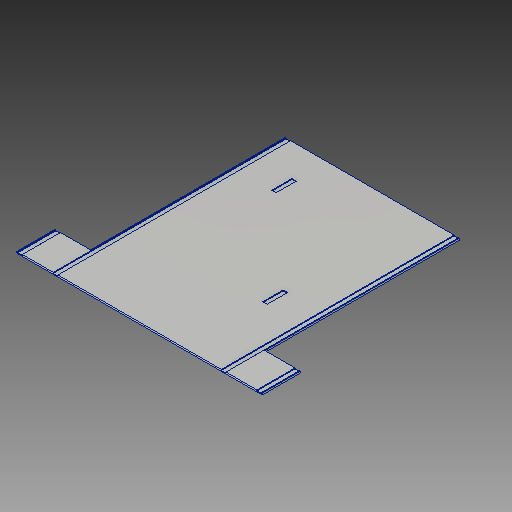
# Autodesk Inventor part: 밑판
Saved by Autodesk Inventor 2017 (Build 210142000, 142)
## iProperties
Part Number: 밑판
Material: 알루미늄 6061
Document SubType Name: Modeling
Designer: minom
Density: 2.7 g/cm^3
Appearance: 알루미늄 - 평지
Mass: 316.314 g
Surface Area: 1244.74 cm^2
Volume: 117.153 cm^3
Author: minom
Autodesk Inventor part; units mm, degrees
ref_plane "YZ Plane" through (0, 0, 0) normal (1, 0, 0) x (0, 1, 0)
ref_plane "XZ Plane" through (0, 0, 0) normal (0, 1, 0) x (-1, 0, 0)
ref_plane "XY Plane" through (0, 0, 0) normal (0, 0, 1) x (1, 0, 0)
sketch "스케치1" plane through (0, 0, 0) normal (0, 1, 0) x (-1, 0, 0)
  line L0 (-43, 66) -> (-249, 66)
  line L1 (-249, 66) -> (-249, -209)
  line L2 (-249, -209) -> (-43, -209)
  line L3 (-43, -209) -> (-43, 66)
  point P0 (0, 0)
  dimension "d0" = 206
  dimension "d1" = 275
  constraints: 8 end point, 2 parallel, 1 horizontal, 1 perpendicular
  measures "d0" distance of L2.end L1.end
  measures "d1" distance of L1.end L0.end
extrude "돌출1" add sketch "스케치1" along normal blind 2
sketch "스케치2" plane through (0, 2, 0) normal (0, 1, 0) x (1, 0, 0)
  line L0 (43, -66) -> (249, -66) projected
  line L1 (249, -66) -> (248, -66)
  line L2 (248, -66) -> (248, 209)
  line L3 (249, 209) -> (43, 209) projected
  line L4 (43, 209) -> (43, -66) projected
  line L5 (43, -66) -> (44, -66)
  line L6 (44, -66) -> (44, 209)
  line L7 (44, 209) -> (49.4, 209)
  line L8 (49.4, 209) -> (49.4, -66)
  line L9 (248, -66) -> (242.6, -66)
  line L10 (242.6, -66) -> (242.6, 209)
  line L11 (49.4, -66) -> (44, -66)
  line L12 (49.4, 209) -> (44, 209)
  point P0 (0, 0)
  dimension "d4" = 1
  dimension "d5" = 5.4
  dimension "d6" = 5.4
  dimension "d9" = 1
  constraints: 20 end point, 6 point on line, 5 perpendicular, 2 collinear
  measures "d4" distance of L0.end L1.end
  measures "d5" distance of L6.end L7.end
  measures "d6" distance of L1.end L9.end
  measures "d9" distance between parallel lines of L6 L4
extrude "돌출2" cut sketch "스케치2" against normal blind 1 contours L6 L3 L8 L0 | L10 L3 L2 L0
sketch "스케치3" plane through (0, 2, 0) normal (0, 1, 0) x (1, 0, 0)
  line L0 (197.8, 27.6733) -> (203, 27.6733)
  line L1 (203, 27.6733) -> (203, 51.8733)
  line L2 (203, 51.8733) -> (197.8, 51.8733)
  line L3 (197.8, 51.8733) -> (197.8, 27.6733)
  point P0 (0, 0)
  dimension "d10" = 5.2
  dimension "d11" = 24.2
  constraints: 8 end point, 2 parallel, 1 horizontal, 1 perpendicular, 1 other
  measures "d10" distance of L0.start L0.end
  measures "d11" distance of L0.end L1.end
extrude "돌출3" cut sketch "스케치3" against normal blind 1
sketch "스케치4" plane through (0, 2, 0) normal (0, 1, 0) x (1, 0, 0)
  line L0 (94.2, 171) -> (89, 171)
  line L1 (89, 171) -> (89, 147)
  line L2 (89, 147) -> (94.2, 147)
  line L3 (94.2, 147) -> (94.2, 171)
  point P0 (0, 0)
  dimension "d14" = 5.2
  constraints: 8 end point, 2 parallel, 1 horizontal, 1 perpendicular, 1 other
  measures "d14" distance of L0.start L0.end
extrude "돌출4" cut sketch "스케치4" against normal blind 1
sketch "스케치5" plane through (0, 0, 0) normal (0, -1, 0) x (1, 0, 0)
  line L0 (43, -209) -> (43, 66) projected
  line L1 (43, 66) -> (1, 66)
  line L2 (1, 66) -> (1, 21)
  line L3 (1, 21) -> (43, 21)
  line L4 (249, 66) -> (291, 66)
  line L5 (291, 66) -> (291, 21)
  line L6 (291, 21) -> (249, 21)
  line L7 (249, 66) -> (249, -209) projected
  point P0 (0, 0)
  dimension "d17" = 42
  dimension "d18" = 45
  dimension "d19" = 42
  dimension "d20" = 45
  constraints: 12 end point, 6 point on line, 2 perpendicular, 1 horizontal
  measures "d17" distance of L0.end L1.end
  measures "d18" distance of L1.end L2.end
  measures "d19" distance of L4.start L4.end
  measures "d20" distance of L4.end L5.end
extrude "돌출5" add sketch "스케치5" against normal blind 2
sketch "스케치6" plane through (0, 2, 0) normal (0, 1, 0) x (1, 0, 0)
  line L0 (44, -66) -> (44, 209) projected
  line L1 (44, 209) -> (43, 209) projected
  line L2 (43, 209) -> (43, -21) projected
  line L3 (43, -21) -> (1, -21) projected
  line L4 (1, -21) -> (1, -66) projected
  line L5 (1, -66) -> (44, -66) projected
  line L6 (248, 209) -> (248, -66) projected
  line L7 (248, -66) -> (291, -66) projected
  line L8 (291, -66) -> (291, -21) projected
  line L9 (291, -21) -> (249, -21) projected
  line L10 (249, -21) -> (249, 209) projected
  line L11 (249, 209) -> (248, 209) projected
  line L12 (2, -66) -> (2, -21)
  line L13 (1, -66) -> (291, -66) projected
  line L14 (7.4, -66) -> (7.4, -21)
  line L15 (248, -66) -> (291, -66) projected
  line L16 (290, -66) -> (290, -21)
  line L17 (284.6, -66) -> (284.6, -21)
  line L18 (291, -21) -> (249, -21) projected
  point P0 (0, 0)
  dimension "d23" = 5.4
  dimension "d24" = 1
  dimension "d25" = 1
  dimension "d26" = 5.4
  constraints: 8 end point, 8 point on line, 3 perpendicular, 1 parallel
  measures "d23" distance between parallel lines of L14 L12
  measures "d24" distance between parallel lines of L12 L4
  measures "d25" distance between parallel lines of L8 L16
  measures "d26" distance between parallel lines of L16 L17
extrude "돌출6" cut sketch "스케치6" against normal blind 1 contours L5 L12 L3 L14 | L17 L9 L16 L7
